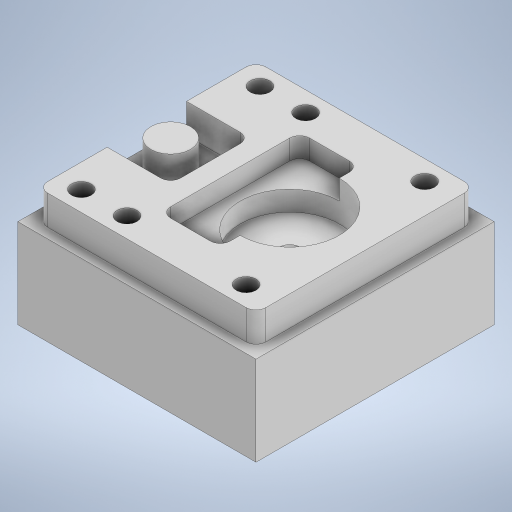
# Autodesk Inventor part: A2P1
Saved by Autodesk Inventor 2023.2 (Build 272271000, 271)
## iProperties
Created: 2023-01-23
Part Number: A2P1
Material: Generic
Document SubType Name: Modeling
Designer: manas
Density: 1 g/cm^3
Appearance: Default
Author: manas
Autodesk Inventor part; units mm, degrees
ref_plane "YZ Plane" through (0, 0, 0) normal (1, 0, 0) x (0, 1, 0)
ref_plane "XZ Plane" through (0, 0, 0) normal (0, 1, 0) x (-1, 0, 0)
ref_plane "XY Plane" through (0, 0, 0) normal (0, 0, 1) x (1, 0, 0)
sketch "Sketch1" plane through (0, 0, 0) normal (0, 1, 0) x (-1, 0, 0)
  line L0 (30, 30) -> (-30, 30)
  line L1 (-30, 30) -> (-30, -30)
  line L2 (-30, -30) -> (30, -30)
  line L3 (30, -30) -> (30, 30)
  line L4 (30, 30) -> (-30, -30) construction
  line L5 (-30, 30) -> (30, -30) construction
  point P0 (0, 0)
  dimension "d0" = 60
  dimension "d1" = 60
  constraints: 12 end point, 2 midpoint, 2 parallel, 1 horizontal, 1 perpendicular
  measures "d0" distance of L2.end L1.end
  measures "d1" distance of L1.end L0.end
extrude "Extrusion1" add sketch "Sketch1" along normal blind 22.5
sketch "Sketch2" plane through (0, 22.5, 0) normal (0, 1, 0) x (1, 0, 0)
  line L0 (-25, 27.5) -> (25, 27.5)
  line L1 (27.5, 25) -> (27.5, -25)
  line L2 (25, -27.5) -> (-25, -27.5)
  line L3 (-27.5, 27.5) -> (27.5, -27.5) construction
  line L4 (27.5, 27.5) -> (-27.5, -27.5) construction
  arc A0 (-27.5, -25) -> (-25, -27.5) centre (-25, -25) ccw
  arc A1 (-25, 27.5) -> (-27.5, 25) centre (-25, 25) ccw
  arc A2 (27.5, 25) -> (25, 27.5) centre (25, 25) ccw
  arc A3 (25, -27.5) -> (27.5, -25) centre (25, -25) ccw
  line L5 (-27.5, -10) -> (-14, -10)
  line L6 (-11.5, -7.5) -> (-11.5, 7.5)
  line L7 (-14, 10) -> (-27.5, 10)
  line L8 (-27.5, -10) -> (-11.5, 10) construction
  line L9 (-11.5, -10) -> (-27.5, 10) construction
  line L10 (30, -30) -> (30, 30) projected
  arc A4 (-14, -10) -> (-11.5, -7.5) centre (-14, -7.5) ccw
  arc A5 (-11.5, 7.5) -> (-14, 10) centre (-14, 7.5) ccw
  line L11 (-27.5, -25) -> (-27.5, -10)
  line L12 (-27.5, 10) -> (-27.5, 25)
  point P0 (0, 0)
  point P1 (-19.5, 0)
  dimension "d4" = 55
  dimension "d5" = 55
  dimension "d6" = 2.5
  dimension "d19" = 16
  dimension "d20" = 20
  dimension "d21" = 41.5
  dimension "d22" = 2.5
  constraints: 24 end point, 14 tangent, 12 point on circle, 10 point on line, 6 centre point, 4 equal radius, 4 midpoint, 4 parallel, 2 horizontal, 2 perpendicular
  measures "d4" distance of L3.end L4.end
  measures "d5" distance of L4.start L3.end
  measures "d6" radius of A0
  measures "d19" distance of L7.end L8.end
  measures "d20" distance of L8.end L9.start
  measures "d21" distance between parallel lines of L10 L6
  measures "d22" radius of A4
extrude "Extrusion2" add sketch "Sketch2" along normal blind 7.5
sketch "Sketch3" plane through (0, 30, 0) normal (0, 1, 0) x (1, 0, 0)
  circle A0 centre (8.5, 0) radius 12.5
  line L0 (30, -30) -> (30, 30) projected
  point P0 (0, 0)
  dimension "d9" = 25
  dimension "d10" = 21.5
  constraints: 1 centre point
  measures "d9" diameter of A0
  measures "d10" distance from line of L0 A0.centre
extrude "Extrusion3" cut sketch "Sketch3" against normal blind 10
sketch "Sketch4" plane through (0, 30, 0) normal (0, 1, 0) x (1, 0, 0)
  line L0 (-4, 17.5) -> (6, 17.5)
  line L1 (8.5, 15) -> (8.5, -15)
  line L2 (6, -17.5) -> (-4, -17.5)
  line L3 (-6.5, -15) -> (-6.5, 15)
  line L4 (-6.5, 17.5) -> (8.5, -17.5) construction
  line L5 (8.5, 17.5) -> (-6.5, -17.5) construction
  line L6 (30, -30) -> (30, 30) projected
  arc A0 (-6.5, -15) -> (-4, -17.5) centre (-4, -15) ccw
  arc A1 (-4, 17.5) -> (-6.5, 15) centre (-4, 15) ccw
  arc A2 (8.5, 15) -> (6, 17.5) centre (6, 15) ccw
  arc A3 (6, -17.5) -> (8.5, -15) centre (6, -15) ccw
  point P0 (0, 0)
  point P1 (1, 0)
  dimension "d13" = 15
  dimension "d14" = 35
  dimension "d15" = 36.5
  dimension "d16" = 2.5
  constraints: 12 end point, 8 point on circle, 8 point on line, 8 tangent, 4 centre point, 3 equal radius, 2 midpoint, 2 parallel, 1 horizontal, 1 perpendicular
  measures "d13" distance of L4.end L5.end
  measures "d14" distance of L5.start L4.end
  measures "d15" distance between parallel lines of L6 L3
  measures "d16" radius of A0
extrude "Extrusion4" cut sketch "Sketch4" against normal blind 5
sketch "Sketch5" plane through (0, 22.5, 0) normal (0, 1, 0) x (1, 0, 0)
  circle A0 centre (-21.5, 0) radius 5
  line L0 (30, -30) -> (30, 30) projected
  point P0 (0, 0)
  dimension "d23" = 10
  dimension "d24" = 51.5
  constraints: 1 centre point
  measures "d23" diameter of A0
  measures "d24" distance from line of L0 A0.centre
extrude "Extrusion5" add sketch "Sketch5" along normal blind 7.5
sketch "Sketch6" plane through (8.5, 20, 0) normal (0, 1, 0) x (1, 0, 0)
  circle A0 centre (0, 0) radius 2.5
  point P0 (-8.5, 0)
  dimension "d27" = 5
  constraints: 1 centre point
  measures "d27" diameter of A0
extrude "Extrusion6" cut sketch "Sketch6" against normal blind 12.5
sketch "Sketch7" plane through (0, 30, 0) normal (0, 1, 0) x (1, 0, 0)
  circle A0 centre (20, -22.5) radius 2.5
  line L0 (30, -30) -> (30, 30) projected
  line L1 (-30, -30) -> (30, -30) projected
  circle A1 centre (20, 22.5) radius 2.5
  circle A2 centre (-10, -22.5) radius 2.5
  circle A3 centre (-10, 22.5) radius 2.5
  circle A4 centre (-21.5, -22.5) radius 2.5
  circle A5 centre (-21.5, 22.5) radius 2.5
  point P0 (0, 0)
  dimension "d30" = 5
  dimension "d31" = 10
  dimension "d32" = 7.5
  dimension "d35" = 45
  dimension "d40" = 5
  dimension "d41" = 40
  dimension "d44" = 45
  dimension "d47" = 11.5
  constraints: 6 centre point, 2 vertical, 1 horizontal, 8 other
  measures "d30" diameter of A0
  measures "d31" distance from line of L0 A0.centre
  measures "d32" distance from line of L1 A0.centre
  measures "d35" distance of A0.centre A1.centre
  measures "d40" diameter of A2
  measures "d41" distance from line of L0 A2.centre
  measures "d44" distance of A2.centre A3.centre
  measures "d47" distance of A2.centre A4.centre
extrude "Extrusion7" cut sketch "Sketch7" against normal blind 10
body "Solid1"
